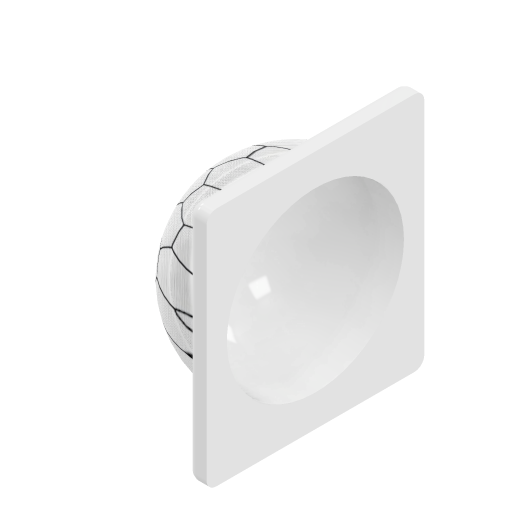
# Autodesk Inventor part: Fresnel
Saved by Autodesk Inventor 2024 (Build 280153000, 153)
## iProperties
Created: 2024-09-23
Part Number: Fresnel
Material: Generic
Document SubType Name: Modeling
Designer: Laith Al-Sadi
Density: 1 g/cm^3
Appearance: White
Author: Laith Al-Sadi
Autodesk Inventor part; units mm, degrees
ref_plane "YZ Plane" through (0, 0, 0) normal (1, 0, 0) x (0, 1, 0)
ref_plane "XZ Plane" through (0, 0, 0) normal (0, 1, 0) x (-1, 0, 0)
sketch "Sketch1" plane through (0, 0, 0) normal (0, 1, 0) x (-1, 0, 0)
  line L0 (0, 0) -> (0, -10)
  arc A0 (0, -10) -> (10, 0) centre (0, 0) ccw
  line L1 (10, 0) -> (0, 0)
  line L2 (1, -1) -> (8.9443, -1)
  arc A1 (1, -8.9443) -> (8.9443, -1) centre (0, 0) ccw
  line L3 (1, -8.9443) -> (1, -1)
  arc A2 (8.9443, -1) -> (9, 0) centre (0, 0) ccw
  line L4 (1, -1) -> (1, 0)
  dimension "d0" = 10
  dimension "d1" = 10
  dimension "d2" = 10
  dimension "d8" = 1
  dimension "d9" = 1
  dimension "d10" = 1
  dimension "d11" = 1
  constraints: 10 end point, 6 point on circle, 3 centre point, 2 point on line, 1 horizontal alignment, 1 perpendicular, 1 tangent, 1 vertical
  measures "d0" distance of L0.start L0.end
  measures "d1" radius of A0
  measures "d2" distance of L0.start L1.start
  measures "d8" radial gap between concentric circles of A0 A1
  measures "d9" distance between parallel lines of L0 L3
  measures "d10" distance between parallel lines of L1 L2
  measures "d11" distance of A2.end L1.start
revolve "Revolution1" add sketch "Sketch1" angle 360 about axis through (-10, 0, 0) along (1, 0, 0) contours L1 L4 L3 A1 A2 A0 L0
sketch "Sketch2" plane through (0, 0, 0) normal (1, 0, 0) x (0, 0, -1)
  line L0 (-11, 12.15) -> (11, 12.15)
  line L1 (11, 12.15) -> (11, -12.15)
  line L2 (11, -12.15) -> (-11, -12.15)
  line L3 (-11, -12.15) -> (-11, 12.15)
  line L4 (-11, 12.15) -> (11, -12.15) construction
  line L5 (11, 12.15) -> (-11, -12.15) construction
  point P0 (0, 0)
  dimension "d4" = 24.3
  dimension "d39" = 22
  constraints: 12 end point, 2 midpoint, 2 parallel, 1 horizontal, 1 perpendicular
  measures "d4" distance of L0.end L1.end
  measures "d39" distance of L0.start L0.end
extrude "Extrusion1" add sketch "Sketch2" along normal blind 2
sketch "Sketch3" plane through (2, 0, 0) normal (1, 0, 0) x (0, 0, -1)
  circle A0 centre (0, 0) radius 10 projected
  circle A1 centre (0, 0) radius 8.9443 projected
extrude "Extrusion2" cut sketch "Sketch3" against normal blind 3 contours A1
fillet "Fillet1" radius 1 8 edges at (1, 12.15, 11) (1, 12.15, -11) (1, -12.15, -11) (1, -12.15, 11) (0, 12.15, 0) (0, 0, 11) (0, -12.15, 0) (0, 0, -11)
ref_plane "Work Plane1" through (-10, 0, 0) normal (-1, 0, 0) x (0, 0, 1)
sketch "Sketch6" plane through (-10, 0, 0) normal (-1, 0, 0) x (0, 0, 1)
  line L0 (-25, 14.1509) -> (25, 14.1509) construction
  line L1 (25, 14.1509) -> (25, -14.1509) construction
  line L2 (25, -14.1509) -> (-25, -14.1509) construction
  line L3 (-25, -14.1509) -> (-25, 14.1509) construction
  point P0 (0, 0)
  point P1 (25, 0)
  point P2 (0, 14.1509)
  dimension "d23" = 50
  constraints: 2 midpoint, 1 horizontal, 1 horizontal alignment, 1 vertical alignment, 2 other
  measures "d23" distance of L0.start L0.end
decal "Decal1"
equation "\"d1\" = d0"
equation "\"d2\" = d0"
body "Solid1"
